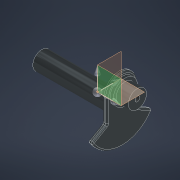
# Autodesk Inventor part: P015-Vilbrequin
Saved by Autodesk Inventor 2021.3 (Build 253353000, 353)
## iProperties
Company: HES-SO
Created: 2022-04-01
Part Number: P015-Vilbrequin
Material: Iron, Gray
Document SubType Name: Modeling
Designer: Rémi & Elise
Density: 7.15 g/cm^3
Appearance: Iron Gray
Mass: 68.6833 g
Surface Area: 45.3336 cm^2
Volume: 9.60606 cm^3
Author: Rémi & Elise
Title: P015 - Vilebrequin
Autodesk Inventor part; units mm, degrees
ref_plane "YZ Plane" through (0, 0, 0) normal (1, 0, 0) x (0, 1, 0)
ref_plane "XZ Plane" through (0, 0, 0) normal (0, 1, 0) x (-1, 0, 0)
ref_plane "XY Plane" through (0, 0, 0) normal (0, 0, 1) x (1, 0, 0)
sketch "Sketch2" plane through (0, 0, 0) normal (1, 0, 0) x (0, 1, 0)
  arc A0 (-19.9186, -11.5) -> (19.9186, -11.5) centre (0, 0) ccw
  line L0 (-19.9186, -11.5) -> (-10, -5.7735)
  line L1 (-10, -5.7735) -> (-10, 9.2265)
  line L2 (19.9186, -11.5) -> (10, -5.7735)
  line L3 (10, -5.7735) -> (10, 9.2265)
  arc A1 (10, 9.2265) -> (-10, 9.2265) centre (0, 9.2265) ccw
  dimension "d1" = 20
  dimension "d2" = 15
  dimension "d3" = 23
  dimension "d54" = 120
  dimension "d55" = 120
  constraints: 8 end point, 4 point on circle, 2 centre point, 2 horizontal alignment, 2 point on line, 1 coincident, 1 vertical, 1 vertical alignment
  measures "d1" distance between parallel lines of L3 L1
  measures "d2" distance of L2.end L3.end
  measures "d3" radius of A0
  measures "d54" angle of L2 L3
  measures "d55" angle of L1 L0
extrude "Extrusion1" add sketch "Sketch2" along normal blind 3
sketch "Sketch10" plane through (0, 0, 0) normal (-1, 0, 0) x (0, 0, 1)
  circle A0 centre (0, 0) radius 6
  dimension "d25" = 12
  constraints: 1 centre point, 1 coincident
  measures "d25" diameter of A0
extrude "Extrusion8" add sketch "Sketch10" along normal blind 50
sketch "Sketch11" plane through (3, 0, 0) normal (1, 0, 0) x (0, 0, -1)
  circle A0 centre (-9.2265, 0) radius 6
  circle A1 centre (-9.2265, 0) radius 8
  arc A2 (11.5, -19.9186) -> (11.5, 19.9186) centre (0, 0) ccw projected
  line L0 (11.5, 19.9186) -> (5.7735, 10) projected
  line L1 (5.7735, 10) -> (-9.2265, 10) projected
  arc A3 (-9.2265, 10) -> (-9.2265, -10) centre (-9.2265, 0) ccw projected
  line L2 (-9.2265, -10) -> (5.7735, -10) projected
  line L3 (5.7735, -10) -> (11.5, -19.9186) projected
  dimension "d29" = 12
  dimension "d32" = 2
  constraints: 2 centre point, 2 coincident, 1 horizontal alignment
  measures "d29" diameter of A0
  measures "d32" radial gap between concentric circles of A1 A0
extrude "Extrusion9" add sketch "Sketch11" along normal blind 10 contours A0
extrude "Extrusion10" add sketch "Sketch11" along normal blind 2 contours A1
sketch "Sketch12" plane through (13, 0, 9.2265) normal (1, 0, 0) x (0, 0, -1)
  circle A0 centre (0, 0) radius 6 construction
  point P0 (9.2265, 0)
  constraints: 1 coincident
hole "Hole2" at (13, 0, 9.2265) direction (-1, 0, 0) diameter 3.242 depth 10 tip angle 118 thread size "M4x0.7" class "6H" standard "ISO Metric profile"
fillet "Fillet3" radius 1 16 edges at (3, 0, -23) (3, 14.9593, -8.6368) (3, 10, 1.7265) (3, 0, 19.2265) (3, -10, 1.7265) (3, -14.9593, -8.6368) (0, 0, -23) (0, -14.9593, -8.6368) (0, -10, 1.7265) (0, 0, 19.2265) (0, 10, 1.7265) (0, 14.9593, -8.6368) (1.5, -10, -5.7735) (1.5, -19.9186, -11.5) (1.5, 10, -5.7735) (1.5, 19.9186, -11.5)
equation "\"d55\" = d54"
body "Solid1"
